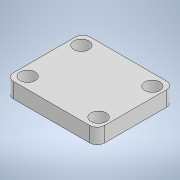
# Autodesk Inventor part: Крепление двигателя2
Saved by Autodesk Inventor 2020 (Build 240168000, 168)
## iProperties
Created: 2021-06-13
Part Number: Крепление двигателя2
Material: Типовые
Document SubType Name: Обычные детали
Designer: Антон
Density: 1 g/cm^3
Appearance: По умолчанию
Sheet Metal Rule: По умолчанию
Author: Антон
Autodesk Inventor part; units mm, degrees
ref_plane "YZ Plane" through (0, 0, 0) normal (1, 0, 0) x (0, 1, 0)
ref_plane "XZ Plane" through (0, 0, 0) normal (0, 1, 0) x (-1, 0, 0)
sketch "Эскиз1" plane through (0, 0, 0) normal (0, 1, 0) x (-1, 0, 0)
  line L0 (0, 0) -> (36, 0)
  line L1 (36, 0) -> (36, -30.3)
  line L2 (36, -30.3) -> (0, -30.3)
  line L3 (0, -30.3) -> (0, 0)
  dimension "d0" = 36
  dimension "d1" = 30.3
  constraints: 8 end point, 2 parallel, 1 horizontal, 1 perpendicular
  measures "d0" distance of L1.end L2.end
  measures "d1" distance of L0.end L1.end
extrude "Выдавливание1" add sketch "Эскиз1" along normal blind 6
sketch "Эскиз2" plane through (0, 6, 0) normal (0, 1, 0) x (1, 0, 0)
  line L0 (-36, 30.3) -> (-36, 0) projected
  line L1 (-36, 0) -> (0, 0) projected
  line L2 (-18, 0) -> (-18, 30.3)
  line L3 (0, 30.3) -> (-36, 30.3) projected
  line L4 (-36, 15.15) -> (0, 15.15)
  line L5 (0, 0) -> (0, 30.3) projected
  point P0 (-32, 4.55)
  point P1 (-32, 25.75)
  point P2 (-4, 4.55)
  point P3 (-4, 25.75)
  point P4 (-32, 4.55)
  dimension "d52" = 14
  dimension "d53" = 10.6
  constraints: 4 end point, 4 midpoint, 3 symmetric about line, 1 coincident
  measures "d52" distance from line of L2 point (-32, 4.55)
  measures "d53" distance from line of L4 point (-32, 4.55)
hole "Отверстие1" at (-32, 6, -4.55) at (-32, 6, -25.75) at (-4, 6, -25.75) at (-4, 6, -4.55) direction (0, -1, 0) diameter 3.2 end through all counterbore diameter 6 counterbore depth 5
sketch "Эскиз4" plane through (0, 0, -2.95) normal (1, 0, 0) x (0, 0, -1)
  line L0 (12.2, 0) -> (12.2, -13.5)
  circle A0 centre (12.2, -13.5) radius 18.5
  line L1 (-2.95, 3) -> (27.35, 3)
  line L2 (-2.95, 0) -> (-2.95, 6) projected
  line L3 (27.35, 0) -> (27.35, 6) projected
  line L4 (-2.95, 0) -> (27.35, 0) projected
  dimension "d27" = 13.5
  dimension "d38" = 37
  constraints: 4 end point, 3 midpoint, 1 centre point, 1 coincident, 1 vertical
  measures "d27" distance of L0.start L0.end
  measures "d38" diameter of A0
ref_plane "РабПлоскость3" through (-8, 0, 0) normal (1, 0, 0) x (0, 0, -1)
ref_plane "РабПлоскость2" through (-18, 0, 0) normal (1, 0, 0) x (0, 0, -1)
extrude "Выдавливание3" cut sketch "Эскиз4" against normal blind 7 from surface at -8 contours A0 L4 | L4 A0 L1 | L1 A0
fillet "Сопряжение3" radius 2.95 4 edges at (-36, 3, 0) (-36, 3, -30.3) (0, 3, 0) (0, 3, -30.3)
equation "\"Радиус_гибки\" = Толщина"
equation "\"Ширина_просечки\" = Толщина"
equation "\"Глубина_просечки\" = 0.5 * Толщина"
equation "\"Размер_просечки\" = 4 * Толщина"
equation "\"Мин_остаток\" = 2 * Толщина"
equation "\"Радиус_перехода\" = Радиус_гибки"
equation "\"Радиус_Якоби\" = Толщина"
equation "\"Размер_зазора\" = Толщина"
equation "\"Толщина\" = 0.5"
